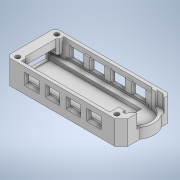
# Autodesk Inventor part: New_case
Saved by Autodesk Inventor 2020 (Build 240168000, 168)
## iProperties
Created: 2022-08-09
Part Number: New_case
Material: Типовые
Document SubType Name: Modeling
Designer: NoName
Density: 1 g/cm^3
Appearance: По умолчанию
Author: NoName
Autodesk Inventor part; units mm, degrees
ref_plane "YZ Plane" through (0, 0, 0) normal (1, 0, 0) x (0, 1, 0)
ref_plane "XZ Plane" through (0, 0, 0) normal (0, 1, 0) x (-1, 0, 0)
ref_plane "XY Plane" through (0, 0, 0) normal (0, 0, 1) x (1, 0, 0)
sketch "Эскиз1" plane through (0, 0, 0) normal (0, 1, 0) x (-1, 0, 0)
  line L0 (-39.8, 8.2) -> (0, 8.2)
  line L1 (0, 8.2) -> (0, -8.2)
  line L2 (0, -8.2) -> (-39.8, -8.2)
  line L3 (-39.8, -8.2) -> (-39.8, 8.2) construction
  arc A0 (-39.8, 4.2) -> (-39.8, -8.2) centre (-39.8, -2) ccw
  line L4 (-39.8, 8.2) -> (-39.8, 4.2)
  arc A1 (-45.8, 2.3313) -> (-45.8, -6.3313) centre (-39.8, -2) ccw
  line L5 (-45.8, -10) -> (1.2, -10)
  line L6 (1.2, -10) -> (1.2, 10)
  line L7 (1.2, 10) -> (-45.8, 10)
  line L8 (-45.8, 10) -> (-45.8, 2.3313)
  line L9 (-45.8, -6.3313) -> (-45.8, -10)
  line L10 (-41.8, 3.8686) -> (-41.8, 5)
  line L11 (-41.8, 5) -> (-39.8, 5)
  point P0 (0, 0)
  point P1 (0, 0)
  point P2 (1.2, 0)
  dimension "d1" = 16.4
  dimension "d2" = 39.8
  dimension "d3" = 6.2
  dimension "d7" = 20
  dimension "d9" = 6
  dimension "d12" = 1.2
  dimension "d20" = 1.2
  dimension "d21" = 5
  dimension "d22" = 2
  constraints: 24 end point, 5 point on circle, 3 horizontal, 3 point on line, 3 vertical, 2 centre point, 2 coincident, 2 midpoint, 2 parallel, 2 perpendicular, 1 collinear, 1 horizontal alignment, 1 vertical alignment
  measures "d1" distance of L0.end L1.end
  measures "d2" distance between parallel lines of L3 L1
  measures "d3" radius of A0
  measures "d7" distance between parallel lines of L7 L5
  measures "d9" distance between parallel lines of L3 L8
  measures "d12" distance between parallel lines of L6 L1
  measures "d20" radial gap between concentric circles of A1 A0
  measures "d21" distance between parallel lines of L7 L11
  measures "d22" distance between parallel lines of L3 L10
extrude "Выдавливание1" add sketch "Эскиз1" along normal blind 6
sketch "Эскиз3" plane through (0, 0, 0) normal (0, -1, 0) x (1, 0, 0)
  line L0 (45.8, -10) -> (-1.2, -10) projected
  arc A0 (45.8, -6.3313) -> (45.8, 2.3313) centre (39.8, -2) ccw projected
  line L1 (45.8, 10) -> (45.8, 2.3313) projected
  line L2 (-1.2, 10) -> (45.8, 10) projected
  line L3 (-1.2, -10) -> (-1.2, 10) projected
  line L4 (39.8, 5) -> (39.8, 8.2) projected
  arc A1 (39.8, -8.2) -> (41.8, 3.8686) centre (39.8, -2) ccw projected
  line L5 (0, -8.2) -> (39.8, -8.2) projected
  line L6 (0, 8.2) -> (0, -8.2) projected
  line L7 (39.8, 8.2) -> (0, 8.2) projected
  line L8 (0, 6.5) -> (37.6, 6.5)
  line L9 (37.6, 6.5) -> (37.6, -6.5)
  line L10 (37.6, -6.5) -> (0, -6.5)
  line L11 (0, -6.5) -> (0, 6.5)
  line L12 (0, 8.2) -> (0, -8.2) projected
  line L13 (45.8, -6.3313) -> (45.8, -10) projected
  line L14 (41.8, 5) -> (39.8, 5) projected
  line L15 (41.8, 3.8686) -> (41.8, 5) projected
  point P0 (0, 0)
  point P1 (0, 0)
  point P2 (0, -6.5)
  dimension "d13" = 13
  dimension "d14" = 37.6
  constraints: 8 end point, 2 midpoint, 2 parallel, 1 horizontal, 1 perpendicular, 1 point on line
  measures "d13" distance between parallel lines of L10 L8
  measures "d14" distance between parallel lines of L11 L9
extrude "Выдавливание2" add sketch "Эскиз3" along normal blind 1.6 contours L0 L3 L2 L1 A0 L13 | L14 L15 A1 L5 L6 L10 L9 L8 L7 L4
sketch "Эскиз4" plane through (0, -1.6, 0) normal (0, -1, 0) x (1, 0, 0)
  line L0 (-1.2, -10) -> (45.8, -10) projected
  arc A0 (45.8, -6.3313) -> (45.8, 2.3313) centre (39.8, -2) ccw projected
  line L1 (45.8, 2.3313) -> (45.8, 10) projected
  line L2 (45.8, 10) -> (-1.2, 10) projected
  line L3 (-1.2, 10) -> (-1.2, -10) projected
  line L4 (37.6, -6.5) -> (0, -6.5) projected
  line L5 (0, -6.5) -> (0, 6.5) projected
  line L6 (0, 6.5) -> (37.6, 6.5) projected
  line L7 (37.6, 6.5) -> (37.6, -6.5) projected
  line L8 (45.8, -10) -> (45.8, -6.3313) projected
  point P0 (0, 0)
extrude "Выдавливание3" add sketch "Эскиз4" along normal blind 0.6 contours L3 L2 L1 A0 L8 L0 | L4 L5 L6 L7
sketch "Эскиз5" plane through (0, 6, 0) normal (0, 1, 0) x (1, 0, 0)
  line L0 (3.6, 8.7) -> (39.8, 8.7)
  line L1 (39.8, 8.7) -> (39.8, -8.7)
  line L2 (39.8, -8.7) -> (3.6, -8.7)
  line L3 (3.6, -8.7) -> (3.6, 8.7)
  line L4 (0, -8.2) -> (0, 8.2) projected
  line L5 (-1.2, 10) -> (-1.2, -10) projected
  line L6 (-1.2, -10) -> (45.8, -10) projected
  line L7 (45.8, -10) -> (45.8, -2.3313) projected
  arc A0 (45.8, -2.3313) -> (45.8, 6.3313) centre (39.8, 2) ccw projected
  line L8 (45.8, 6.3313) -> (45.8, 10) projected
  line L9 (45.8, 10) -> (-1.2, 10) projected
  line L10 (0, -8.2) -> (0, 8.2) projected
  line L11 (0, 8.2) -> (39.8, 8.2) projected
  arc A1 (41.8, -3.8686) -> (39.8, 8.2) centre (39.8, 2) ccw projected
  line L12 (41.8, -3.8686) -> (41.8, -5) projected
  line L13 (41.8, -5) -> (39.8, -5) projected
  line L14 (39.8, -5) -> (39.8, -8.2) projected
  line L15 (39.8, -8.2) -> (0, -8.2) projected
  point P0 (0, 0)
  point P1 (3.6, 0)
  point P2 (0, 0)
  point P3 (39.8, -5)
  point P4 (3.6, -8.2)
  point P5 (3.6, 8.2)
  dimension "d23" = 36.2
  dimension "d24" = 17.4
  constraints: 8 end point, 2 midpoint, 2 parallel, 1 horizontal, 1 horizontal alignment, 1 perpendicular, 1 vertical alignment
  measures "d23" distance between parallel lines of L1 L3
  measures "d24" distance of L2.end L0.start
extrude "Выдавливание4" add sketch "Эскиз5" along normal blind 1.6
ref_plane "РабПлоскость1" through (0, 2, 0) normal (0, 1, 0) x (1, 0, 0)
sketch "Эскиз6" plane through (0, 2, 0) normal (0, 1, 0) x (1, 0, 0)
  arc A0 (41.8, -3.8686) -> (39.8, 8.2) centre (39.8, 2) ccw projected
  arc A1 (45.8, -2.3313) -> (45.8, 6.3313) centre (39.8, 2) ccw projected
  arc A2 (45.8, 7.2915) -> (44.0143, 8.8) centre (39.8, 2) ccw
  line L0 (45.8, 10) -> (45.8, 6.3313) projected
  line L1 (45.8, -2.3313) -> (45.8, -10) projected
  arc A3 (43.673, -5) -> (45.8, -3.2915) centre (39.8, 2) ccw
  arc A4 (45.8, -3.2915) -> (45.8, 7.2915) centre (39.8, 2) ccw construction
  line L2 (0, 8.2) -> (39.8, 8.2) projected
  line L3 (41.8, 7.8686) -> (41.8, 8.8)
  line L4 (41.8, 8.8) -> (44.0143, 8.8)
  line L5 (41.8, -3.8686) -> (41.8, -5) projected
  line L6 (41.8, -5) -> (43.673, -5)
  line L7 (43.673, -5) -> (43.673, -6)
  line L8 (43.673, -6) -> (42.373, -6)
  line L9 (42.373, -6) -> (42.373, -4.9788)
  line L10 (45.5131, 7.6) -> (45.8, 7.6)
  line L11 (45.5131, -3.6) -> (45.8, -3.6)
  point P0 (0, 0)
  point P1 (42.373, -5)
  dimension "d28" = 8
  dimension "d29" = 0.6
  dimension "d49" = 1.3
  dimension "d50" = 1
  dimension "d72" = 11.2
  constraints: 16 end point, 9 point on circle, 4 perpendicular, 4 point on line, 3 centre point, 3 coincident, 2 vertical, 1 horizontal, 1 parallel, 1 vertical alignment
  measures "d28" radius of A2
  measures "d29" distance from line of L2 L4.end
  measures "d49" distance between parallel lines of L9 L7
  measures "d50" distance between parallel lines of L6 L8
  measures "d72" distance between parallel lines of L11 L10
extrude "Выдавливание5" cut sketch "Эскиз6" along normal through all
ref_plane "РабПлоскость2" through (0, 2, 0) normal (0, 1, 0) x (1, 0, 0)
sketch "Эскиз7" plane through (0, 2, 0) normal (0, 1, 0) x (1, 0, 0)
  line L0 (0, 6.5) -> (0, -6.5) construction
  line L1 (2.8, -6.2) -> (0, -6.2)
  line L2 (0, -6.2) -> (0, 6.2) construction
  line L3 (0, 6.2) -> (2.8, 6.2)
  line L4 (2.8, 6.2) -> (2.8, -6.2) construction
  line L5 (0, -8.2) -> (0, 8.2) construction
  line L6 (-1.2, 10) -> (-1.2, -10) projected
  line L7 (3.6, 8.2) -> (39.8, 8.2) projected
  line L8 (3.6, 8.2) -> (3.6, 7)
  line L9 (3.6, 7) -> (2.8, 6.2)
  line L10 (39.8, -8.2) -> (0, -8.2) projected
  line L11 (3.6, -8.2) -> (3.6, -7)
  line L12 (3.6, -7) -> (2.8, -6.2)
  line L13 (3.6, -8.2) -> (0, -8.2)
  line L14 (0, -6.2) -> (0, -8.2)
  line L15 (0, 6.2) -> (0, 8.2)
  line L16 (0, 8.2) -> (39.8, 8.2) construction
  line L17 (3.6, 8.2) -> (0, 8.2)
  point P0 (0, 0)
  point P1 (0, 0)
  dimension "d33" = 12.4
  dimension "d34" = 4
  constraints: 24 end point, 3 collinear, 3 perpendicular, 3 point on line, 3 vertical, 2 midpoint, 2 parallel, 1 horizontal
  measures "d33" distance between parallel lines of L1 L3
  measures "d34" distance between parallel lines of L6 L4
extrude "Выдавливание6" add sketch "Эскиз7" along normal up to surface (5.6 mm away)
sketch "Эскиз8" plane through (-1.2, -2.2, -10) normal (-1, 0, 0) x (0, 0, 1)
  line L0 (3.9, 5.7) -> (16.1, 5.7)
  line L1 (16.1, 5.7) -> (16.1, 1)
  line L2 (16.1, 1) -> (3.9, 1)
  line L3 (3.9, 1) -> (3.9, 5.7)
  line L4 (20, 0) -> (0, 0) projected
  line L5 (18.2, 2.2) -> (16.5, 2.2) projected
  line L6 (15, 2.2) -> (18.2, 2.2) projected
  line L7 (13.8686, 2.2) -> (15, 2.2) projected
  line L8 (1.8, 2.2) -> (13.8686, 2.2) projected
  line L9 (3.5, 2.2) -> (1.8, 2.2) projected
  line L10 (16.5, 2.2) -> (3.5, 2.2) projected
  point P0 (10, 2.2)
  point P1 (10, 1)
  point P2 (10, 0)
  dimension "d38" = 4.7
  dimension "d39" = 12.2
  dimension "d41" = 1.2
  constraints: 8 end point, 2 midpoint, 2 parallel, 1 horizontal, 1 perpendicular, 1 vertical alignment
  measures "d38" distance between parallel lines of L2 L0
  measures "d39" distance between parallel lines of L1 L3
  measures "d41" distance between parallel lines of L8 L2
extrude "Выдавливание7" cut sketch "Эскиз8" against normal blind 10
sketch "Эскиз9" plane through (-1.2, 3.5, -6.1) normal (0, -1, 0) x (1, 0, 0)
  line L0 (1.2, 12.3) -> (1.2, -0.1) projected
  line L1 (1.2, 12.3) -> (4, 12.3) projected
  line L2 (1.2, -0.1) -> (4, -0.1)
  line L3 (4, -0.1) -> (4, 12.3)
  line L4 (4, 12.3) -> (1.2, 12.3)
  line L5 (1.2, 12.3) -> (1.2, -0.1)
  point P0 (1.2, 6.1)
  constraints: 8 end point, 2 parallel, 1 coincident, 1 horizontal, 1 perpendicular, 1 point on line
extrude "Выдавливание8" add sketch "Эскиз9" against normal up to surface (4.1 mm away)
chamfer "Фаска1" distance 1 angle 45 1 edges at (2.8, 3.5, 0)
sketch "Эскиз11" plane through (0, 7.6, 0) normal (0, 1, 0) x (1, 0, 0)
  line L0 (-1.2, 10) -> (-1.2, -10) projected
  line L1 (-1.2, 0) -> (45.6686, 0)
  arc A0 (41.8, -3.8686) -> (39.8, 8.2) centre (39.8, 2) ccw projected
  line L2 (45.8, -10) -> (45.8, -3.6) projected
  line L3 (3.6, -8.7) -> (3.6, -7) projected
  line L4 (39.8, -5) -> (39.8, -8.7) projected
  point P0 (0, 0)
  point P1 (1.4, -8)
  point P2 (42, -8)
  point P3 (1.4, 8)
  point P4 (45.8, -3.2915)
  dimension "d58" = 16
  dimension "d67" = 2.2
  dimension "d68" = 2.2
  constraints: 2 end point, 1 horizontal, 1 horizontal alignment, 1 midpoint, 1 point on circle, 1 symmetric about line, 1 vertical alignment
  measures "d58" distance of point (1.4, 8) point (1.4, -8)
  measures "d67" distance from line of point (1.4, -8) L3
  measures "d68" distance from line of L4 point (42, -8)
hole "Отверстие1" at (1.4, 7.6, 8) at (42, 7.6, 8) at (1.4, 7.6, -8) direction (0, -1, 0) diameter 1.9 depth 7.6
chamfer "Фаска2" distance 1.4 angle 45 2 edges at (-1.2, 2.7, 10) (-1.2, 2.7, -10)
chamfer "Фаска3" distance 2.6 angle 45 1 edges at (45.8, 2.7, 10)
chamfer "Фаска4" distance 1 angle 45 1 edges at (45.8, 2.7, -10)
sketch "Эскиз12" plane through (0.2, -2.2, 10) normal (0, 0, 1) x (1, 0, 0)
  line L0 (6, 3.2) -> (12, 3.2)
  line L1 (12, 3.2) -> (12, 7.8)
  line L2 (12, 7.8) -> (6, 7.8)
  line L3 (6, 7.8) -> (6, 3.2)
  line L4 (14.5, 3.2) -> (20.5, 3.2)
  line L5 (20.5, 3.2) -> (20.5, 7.8)
  line L6 (20.5, 7.8) -> (14.5, 7.8)
  line L7 (14.5, 7.8) -> (14.5, 3.2)
  line L8 (23, 3.2) -> (29, 3.2)
  line L9 (29, 3.2) -> (29, 7.8)
  line L10 (29, 7.8) -> (23, 7.8)
  line L11 (23, 7.8) -> (23, 3.2)
  line L12 (31.5, 3.2) -> (37.5, 3.2)
  line L13 (37.5, 3.2) -> (37.5, 7.8)
  line L14 (37.5, 7.8) -> (31.5, 7.8)
  line L15 (31.5, 7.8) -> (31.5, 3.2)
  line L16 (43, 0) -> (0, 0) projected
  line L17 (0, 0) -> (0, 9.8) projected
  line L18 (-1.4, 9.8) -> (-1.4, 0) projected
  line L19 (39.6, 2.2) -> (2.1287, 2.2) projected
  line L20 (41.6, 2.2) -> (39.6, 2.2) projected
  line L21 (39.6, 2.2) -> (41.6, 2.2) projected
  line L22 (2.1287, 2.2) -> (39.6, 2.2) projected
  line L23 (0.2713, 2.2) -> (2.1287, 2.2) projected
  line L24 (-0.2, 2.2) -> (0.2713, 2.2) projected
  line L25 (37.4, 2.2) -> (-0.2, 2.2) projected
  line L26 (-0.2, 2.2) -> (37.4, 2.2) projected
  line L27 (0.2713, 2.2) -> (-0.2, 2.2) projected
  line L28 (2.1287, 2.2) -> (0.2713, 2.2) projected
  point P0 (-0.2, 2.2)
  point P1 (9, 7.8)
  point P2 (3.4, 8.2)
  point P3 (39.6, 8.2)
  dimension "d75" = 8.5
  dimension "d80" = 6
  dimension "d87" = 10.4
  dimension "d88" = 1
  dimension "d94" = 4.6
  constraints: 32 end point, 2 horizontal, 2 parallel, 1 collinear, 1 midpoint, 1 perpendicular, 23 other
  measures "d75" distance of L0.start L4.start
  measures "d80" distance between parallel lines of L1 L3
  measures "d87" distance from line of L18 point (9, 7.8)
  measures "d88" distance between parallel lines of L0 L26
  measures "d94" distance of L2.end L0.start
extrude "Выдавливание9" cut sketch "Эскиз12" against normal through all
sketch "Эскиз13" plane through (39.8, 0, -8.2) normal (0, 0, 1) x (1, 0, 0)
  line L0 (-16.6, 1) -> (-16.6, 5.6) projected
  line L1 (-36.2, 6) -> (0, 6) projected
  line L2 (-19.1, 5.6) -> (-19.1, 1) projected
  line L3 (-19.1, 1) -> (-25.1, 1) projected
  line L4 (-25.1, 1) -> (-25.1, 5.6) projected
  line L5 (-27.6, 5.6) -> (-27.6, 1) projected
  line L6 (-27.6, 1) -> (-33.6, 1) projected
  line L7 (-33.6, 1) -> (-33.6, 5.6) projected
  line L8 (-36.2, 6) -> (-36.2, 2) projected
  line L9 (-36.2, 2) -> (-37.4713, 2) projected
  line L10 (-37.4713, 2) -> (-37.4713, 0) projected
  line L11 (-37.4713, 0) -> (0, 0) projected
  line L12 (0, 0) -> (0, 6) projected
  line L13 (-2.1, 5.6) -> (-2.1, 1) projected
  line L14 (-2.1, 1) -> (-8.1, 1) projected
  line L15 (-8.1, 1) -> (-8.1, 5.6) projected
  line L16 (-10.6, 5.6) -> (-10.6, 1) projected
  line L17 (-10.6, 1) -> (-16.6, 1) projected
  line L18 (-34.8, 0) -> (-0.9, 0)
  line L19 (-0.9, 0) -> (-0.9, 1.4)
  line L20 (-0.9, 1.4) -> (-34.8, 1.4)
  line L21 (-34.8, 1.4) -> (-34.8, 0)
  line L22 (-16.6, 5.6) -> (-10.6, 5.6) projected
  line L23 (-25.1, 5.6) -> (-19.1, 5.6) projected
  line L24 (-8.1, 5.6) -> (-2.1, 5.6) projected
  line L25 (-33.6, 5.6) -> (-27.6, 5.6) projected
  line L26 (-33.6, 5.6) -> (-33.6, 1) projected
  line L27 (0, 6) -> (-36.2, 6) projected
  line L28 (-33.6, 5.6) -> (-27.6, 5.6)
  line L29 (-27.6, 5.6) -> (-27.6, 6)
  line L30 (-27.6, 6) -> (-33.6, 6)
  line L31 (-33.6, 6) -> (-33.6, 5.6)
  line L32 (-25.1, 5.6) -> (-25.1, 1) projected
  line L33 (-25.1, 5.6) -> (-19.1, 5.6)
  line L34 (-19.1, 5.6) -> (-19.1, 6)
  line L35 (-19.1, 6) -> (-25.1, 6)
  line L36 (-25.1, 6) -> (-25.1, 5.6)
  line L37 (-10.6, 5.6) -> (-16.6, 5.6) projected
  line L38 (-16.6, 5.6) -> (-10.6, 5.6)
  line L39 (-10.6, 5.6) -> (-10.6, 6)
  line L40 (-10.6, 6) -> (-16.6, 6)
  line L41 (-16.6, 6) -> (-16.6, 5.6)
  line L42 (-8.1, 5.6) -> (-8.1, 1) projected
  line L43 (-8.1, 5.6) -> (-2.1, 5.6)
  line L44 (-2.1, 5.6) -> (-2.1, 6)
  line L45 (-2.1, 6) -> (-8.1, 6)
  line L46 (-8.1, 6) -> (-8.1, 5.6)
  point P0 (-39.8, 0)
  point P1 (-33.6, 1.4)
  point P2 (-2.1, 1.4)
  point P3 (-8.1, 1.4)
  point P4 (-10.6, 1.4)
  point P5 (-16.6, 1.4)
  point P6 (-19.1, 1.4)
  point P7 (-25.1, 1.4)
  point P8 (-27.6, 1.4)
  dimension "d89" = 1.4
  dimension "d90" = 1.2
  dimension "d91" = 1.2
  constraints: 40 end point, 10 parallel, 5 horizontal, 5 perpendicular, 5 point on line
  measures "d89" distance between parallel lines of L11 L20
  measures "d90" distance between parallel lines of L7 L21
  measures "d91" distance between parallel lines of L13 L19
extrude "Выдавливание10" cut sketch "Эскиз13" against normal blind 0.5 contours L17 L16 L20 L15 L14 L13 L19 L11 L21 L7 L6 L5 L4 L3 L2 L0 | L41 L1 L39 L22 | L23 L36 L1 L34 | L46 L1 L44 L24 | L25 L31 L1 L29
